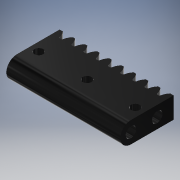
# Autodesk Inventor part: GA04
Saved by Autodesk Inventor 2017 (Build 210142000, 142)
## iProperties
Created: 2018-10-24
Part Number: GA04
Material: ABS Plastic
Document SubType Name: Modeling
Designer: Dell
Density: 1.06 g/cm^3
Appearance: Smooth - Black
Author: Dell
Autodesk Inventor part; units mm, degrees
ref_plane "YZ Plane" through (0, 0, 0) normal (1, 0, 0) x (0, 1, 0)
ref_plane "XZ Plane" through (0, 0, 0) normal (0, 1, 0) x (-1, 0, 0)
ref_plane "XY Plane" through (0, 0, 0) normal (0, 0, 1) x (1, 0, 0)
sketch "Sketch1" plane through (0, 0, 0) normal (0, 0, 1) x (1, 0, 0)
  spline S0 degree 3 poles (-2.7752, 20.8158) (-2.7042, 20.7277) (-2.562, 20.5515) (-2.36, 20.2785) (-2.1667, 19.9993) (-1.9839, 19.7131) (-1.8126, 19.4198) (-1.654, 19.1195) (-1.5101, 18.8118) (-1.3833, 18.4967) (-1.2955, 18.2274) (-1.2397, 18.008) (-1.2095, 17.8408) (-1.1935, 17.6716) (-1.162, 17.5046) (-1.1186, 17.3404) (-1.0623, 17.18) (-0.9883, 17.0268) (-0.8958, 16.884) (-0.7836, 16.7557) (-0.6724, 16.6674) (-0.5769, 16.6065) (-0.4998, 16.5707) (-0.4208, 16.5391) (-0.3383, 16.5188) (-0.2547, 16.503) (-0.1414, 16.4982) (0, 16.5012) (0.1414, 16.4982) (0.2547, 16.503) (0.3383, 16.5188) (0.4208, 16.5391) (0.4998, 16.5707) (0.5769, 16.6065) (0.6724, 16.6674) (0.7836, 16.7557) (0.8958, 16.884) (0.9883, 17.0268) (1.0623, 17.18) (1.1186, 17.3404) (1.162, 17.5046) (1.1935, 17.6716) (1.2095, 17.8408) (1.2397, 18.008) (1.2955, 18.2274) (1.3833, 18.4967) (1.5101, 18.8118) (1.654, 19.1195) (1.8126, 19.4198) (1.9839, 19.7131) (2.1667, 19.9993) (2.36, 20.2785) (2.562, 20.5515) (2.7042, 20.7277) (2.7752, 20.8158) knots 0 0 0 0 0.033953 0.067907 0.10186 0.135813 0.169766 0.203718 0.237669 0.271619 0.305565 0.322541 0.339512 0.356488 0.373464 0.390436 0.407409 0.424381 0.44135 0.458313 0.475267 0.483756 0.492243 0.500732 0.509218 0.517706 0.526192 0.543169 0.560147 0.568632 0.577121 0.585607 0.594095 0.602582 0.611072 0.628025 0.644989 0.661958 0.67893 0.695903 0.712875 0.729851 0.746827 0.763798 0.780774 0.81472 0.84867 0.882621 0.916573 0.950526 0.984479 1.018432 1.052385 1.086339 1.086339 1.086339 1.086339
  circle A0 centre (0, 0) radius 16.5 construction
  circle A1 centre (0, 0) radius 17.8542 construction
  circle A2 centre (0, 0) radius 19 construction
  circle A3 centre (0, 0) radius 21 construction
  line L0 (-2.7752, 20.8158) -> (2.7752, 20.8158)
  point P0 (-2.5639, 20.5501)
  point P1 (-2.3614, 20.2775)
  point P2 (-2.1684, 19.9981)
  point P3 (-1.9858, 19.7119)
  point P4 (-1.8147, 19.4186)
  point P5 (-1.6565, 19.1183)
  point P6 (-1.513, 18.8106)
  point P7 (-1.3869, 18.4953)
  point P8 (-1.2828, 18.1722)
  point P9 (-1.2417, 18.0075)
  point P10 (-1.2119, 17.8405)
  point P11 (-1.1909, 17.672)
  point P12 (-1.16, 17.5051)
  point P13 (-1.1164, 17.341)
  point P14 (-1.0594, 17.1812)
  point P15 (-0.9852, 17.0285)
  point P16 (-0.8925, 16.8864)
  point P17 (-0.78, 16.7594)
  point P18 (-0.648, 16.653)
  point P19 (-0.576, 16.6082)
  point P20 (-0.4995, 16.5714)
  point P21 (-0.4202, 16.541)
  point P22 (-0.3381, 16.5195)
  point P23 (-0.2545, 16.505)
  point P24 (-0.1698, 16.5)
  point P25 (0, 16.5)
  point P26 (0.1698, 16.5)
  point P27 (0.2545, 16.505)
  point P28 (0.3381, 16.5195)
  point P29 (0.4202, 16.541)
  point P30 (0.4995, 16.5714)
  point P31 (0.576, 16.6082)
  point P32 (0.648, 16.653)
  point P33 (0.78, 16.7594)
  point P34 (0.8925, 16.8864)
  point P35 (0.9852, 17.0285)
  point P36 (1.0594, 17.1812)
  point P37 (1.1164, 17.341)
  point P38 (1.16, 17.5051)
  point P39 (1.1909, 17.672)
  point P40 (1.2119, 17.8405)
  point P41 (1.2417, 18.0075)
  point P42 (1.2828, 18.1722)
  point P43 (1.3869, 18.4953)
  point P44 (1.513, 18.8106)
  point P45 (1.6565, 19.1183)
  point P46 (1.8147, 19.4186)
  point P47 (1.9858, 19.7119)
  point P48 (2.1684, 19.9981)
  point P49 (2.3614, 20.2775)
  point P50 (2.5639, 20.5501)
  constraints: 4 centre point, 2 end point, 2 point on circle, 1 horizontal, 111 other
sketch "Sketch2" plane through (0, 0, 0) normal (0, 0, 1) x (1, 0, 0)
  line L0 (32.5, 20.8158) -> (-32.5, 20.8158)
  line L1 (-32.5, 20.8158) -> (-32.5, 14.8158)
  line L2 (-32.5, 14.8158) -> (32.5, 14.8158)
  line L3 (32.5, 14.8158) -> (32.5, 20.8158)
  circle A0 centre (0, 0) radius 21 construction
  point P0 (0, 20.8158)
  point P1 (-2.7752, 20.8158)
  point P2 (2.7752, 20.8158)
  dimension "d2" = 6
  dimension "d3" = 65
  constraints: 8 end point, 2 parallel, 1 horizontal, 1 midpoint, 1 perpendicular, 1 point on line, 1 vertical alignment
  measures "d2" distance of L0.end L1.end
  measures "d3" distance of L1.end L2.end
extrude "Extrusion2" add sketch "Sketch2" along normal blind 10
extrude "Extrusion3" cut sketch "Sketch1" along normal blind 10
pattern_linear "Rectangular Pattern1" count 9 spacing 6.9446 along (-1, 0, 0) of "Extrusion3" first direction both ways yes
sketch "Sketch3" plane through (-32.5, 14.8158, 0) normal (-1, 0, 0) x (0, 0, 1)
  circle A0 centre (5, -3.3166) radius 6
  line L0 (0, 0) -> (10, 0) projected
  point P0 (0, -14.8158)
  point P1 (5, 0)
  dimension "d11" = 12
  constraints: 2 point on circle, 1 centre point, 1 midpoint, 1 vertical alignment
  measures "d11" diameter of A0
extrude "Extrusion4" add sketch "Sketch3" against normal blind 65 contours A0 L0 picked at (5.1596, -3.0992)
sketch "Sketch6" plane through (32.5, 20.8158, 10) normal (1, 0, 0) x (0, 0, -1)
  circle A0 centre (5, -24.3166) radius 6
  arc A1 (0, -6) -> (10, -6) centre (5, -9.3166) ccw projected
  line L0 (-1, -24.3166) -> (-1, -9.3166)
  line L1 (11, -9.3166) -> (11, -24.3166)
  arc A2 (-1, -9.3166) -> (11, -9.3166) centre (5, -9.3166) ccw
  point P0 (10, -20.8158)
  dimension "d21" = 15
  dimension "d22" = 12
  constraints: 6 point on circle, 4 end point, 4 tangent, 2 centre point, 1 concentric, 1 vertical alignment
  measures "d21" distance of A1.centre A0.centre
  measures "d22" diameter of A0
extrude "Extrusion6" add sketch "Sketch6" against normal blind 65
sketch "Sketch7" plane through (32.5, 20.8158, 10) normal (1, 0, 0) x (0, 0, -1)
  arc A0 (-1, -24.3166) -> (11, -24.3166) centre (5, -24.3166) ccw projected
  arc A1 (0, -6) -> (-1, -9.3166) centre (5, -9.3166) ccw projected
  circle A2 centre (5, -24.3166) radius 3
  circle A3 centre (5, -9.3166) radius 3
  point P0 (10, -20.8158)
  dimension "d25" = 6
  dimension "d26" = 6
  constraints: 2 centre point, 2 coincident
  measures "d25" diameter of A2
  measures "d26" diameter of A3
extrude "Extrusion7" cut sketch "Sketch7" against normal through all
sketch "Sketch8" plane through (32.5, -3.5008, 11) normal (0, 0, 1) x (1, 0, 0)
  line L0 (-65, 12) -> (-65, 18) projected
  line L1 (0, 18) -> (0, 12) projected
  line L2 (-65, -3) -> (-65, 3) projected
  line L3 (0, 3) -> (0, -3) projected
  circle A0 centre (-60, 7.5) radius 2.5
  circle A1 centre (-5, 7.5) radius 2.5
  circle A2 centre (-32.5, 7.5) radius 2.5
  line L4 (-5, 7.5) -> (-60, 7.5) construction
  line L5 (0, -6) -> (-65, -6) projected
  line L6 (-65, 3) -> (-65, 12)
  point P0 (-32.5, 3.5008)
  point P1 (-32.5, -6)
  point P2 (-65, 7.5)
  dimension "d29" = 5
  dimension "d30" = 5
  dimension "d31" = 5
  dimension "d32" = 55
  constraints: 4 end point, 3 centre point, 3 midpoint, 1 coincident, 1 horizontal, 1 horizontal alignment, 1 vertical, 1 vertical alignment
  measures "d29" diameter of A0
  measures "d30" diameter of A1
  measures "d31" diameter of A2
  measures "d32" distance of L4.start L4.end
extrude "Extrusion8" cut sketch "Sketch8" against normal through all
sketch "Sketch9" plane through (0, 0, 10) normal (0, 0, 1) x (1, 0, 0)
  spline S0 degree 3 poles (-25.0031, 20.8158) (-25.0741, 20.7277) (-25.2163, 20.5515) (-25.4183, 20.2785) (-25.6116, 19.9993) (-25.7944, 19.7131) (-25.9657, 19.4198) (-26.1243, 19.1195) (-26.2682, 18.8118) (-26.395, 18.4967) (-26.4828, 18.2274) (-26.5386, 18.008) (-26.5688, 17.8408) (-26.5848, 17.6716) (-26.6163, 17.5046) (-26.6597, 17.3404) (-26.716, 17.18) (-26.79, 17.0268) (-26.8825, 16.884) (-26.9947, 16.7557) (-27.1059, 16.6674) (-27.2014, 16.6065) (-27.2785, 16.5707) (-27.3575, 16.5391) (-27.44, 16.5188) (-27.5236, 16.503) (-27.6369, 16.4982) (-27.7783, 16.5012) (-27.9197, 16.4982) (-28.033, 16.503) (-28.1166, 16.5188) (-28.1991, 16.5391) (-28.2781, 16.5707) (-28.3552, 16.6065) (-28.4507, 16.6674) (-28.5619, 16.7557) (-28.6741, 16.884) (-28.7666, 17.0268) (-28.8406, 17.18) (-28.8969, 17.3404) (-28.9403, 17.5046) (-28.9718, 17.6716) (-28.9878, 17.8408) (-29.018, 18.008) (-29.0738, 18.2274) (-29.1616, 18.4967) (-29.2884, 18.8118) (-29.4323, 19.1195) (-29.5909, 19.4198) (-29.7622, 19.7131) (-29.945, 19.9993) (-30.1383, 20.2785) (-30.3403, 20.5515) (-30.4824, 20.7277) (-30.5535, 20.8158) knots 0 0 0 0 0.031255 0.06251 0.093765 0.125019 0.156273 0.187527 0.21878 0.250031 0.28128 0.296906 0.312529 0.328155 0.343782 0.359405 0.375029 0.390652 0.406273 0.421888 0.437494 0.445309 0.453121 0.460935 0.468747 0.476561 0.484372 0.5 0.515628 0.523439 0.531253 0.539065 0.546879 0.554691 0.562506 0.578112 0.593727 0.609348 0.624971 0.640595 0.656218 0.671845 0.687471 0.703094 0.71872 0.749969 0.78122 0.812473 0.843727 0.874981 0.906235 0.93749 0.968745 1 1 1 1 projected
  line L0 (-30.5535, 20.8158) -> (-32.5, 20.8158) projected
  line L1 (-32.5, 20.8158) -> (-32.5, 14.8158) projected
  line L2 (-32.5, 14.8158) -> (32.5, 14.8158) projected
  line L3 (32.5, 14.8158) -> (32.5, 20.8158) projected
  line L4 (32.5, 20.8158) -> (30.5535, 20.8158) projected
  spline S1 degree 3 poles (30.5535, 20.8158) (30.4824, 20.7277) (30.3403, 20.5515) (30.1383, 20.2785) (29.945, 19.9993) (29.7622, 19.7131) (29.5909, 19.4198) (29.4323, 19.1195) (29.2884, 18.8118) (29.1616, 18.4967) (29.0738, 18.2274) (29.018, 18.008) (28.9878, 17.8408) (28.9718, 17.6716) (28.9403, 17.5046) (28.8969, 17.3404) (28.8406, 17.18) (28.7666, 17.0268) (28.6741, 16.884) (28.5619, 16.7557) (28.4507, 16.6674) (28.3552, 16.6065) (28.2781, 16.5707) (28.1991, 16.5391) (28.1166, 16.5188) (28.033, 16.503) (27.9197, 16.4982) (27.7783, 16.5012) (27.6369, 16.4982) (27.5236, 16.503) (27.44, 16.5188) (27.3575, 16.5391) (27.2785, 16.5707) (27.2014, 16.6065) (27.1059, 16.6674) (26.9947, 16.7557) (26.8825, 16.884) (26.79, 17.0268) (26.716, 17.18) (26.6597, 17.3404) (26.6163, 17.5046) (26.5848, 17.6716) (26.5688, 17.8408) (26.5386, 18.008) (26.4828, 18.2274) (26.395, 18.4967) (26.2682, 18.8118) (26.1243, 19.1195) (25.9657, 19.4198) (25.7944, 19.7131) (25.6116, 19.9993) (25.4183, 20.2785) (25.2163, 20.5515) (25.0741, 20.7277) (25.0031, 20.8158) knots 0 0 0 0 0.031255 0.06251 0.093765 0.125019 0.156273 0.187527 0.21878 0.250031 0.28128 0.296906 0.312529 0.328155 0.343782 0.359405 0.375029 0.390652 0.406273 0.421888 0.437494 0.445309 0.453121 0.460935 0.468747 0.476561 0.484372 0.5 0.515628 0.523439 0.531253 0.539065 0.546879 0.554691 0.562506 0.578112 0.593727 0.609348 0.624971 0.640595 0.656218 0.671845 0.687471 0.703094 0.71872 0.749969 0.78122 0.812473 0.843727 0.874981 0.906235 0.93749 0.968745 1 1 1 1 projected
  line L5 (25.0031, 20.8158) -> (23.6089, 20.8158) projected
  spline S2 degree 3 poles (23.6089, 20.8158) (23.5379, 20.7277) (23.3958, 20.5515) (23.1937, 20.2785) (23.0004, 19.9993) (22.8177, 19.7131) (22.6463, 19.4198) (22.4877, 19.1195) (22.3438, 18.8118) (22.2171, 18.4967) (22.1292, 18.2274) (22.0734, 18.008) (22.0432, 17.8408) (22.0272, 17.6716) (21.9957, 17.5046) (21.9523, 17.3404) (21.896, 17.18) (21.822, 17.0268) (21.7296, 16.884) (21.6173, 16.7557) (21.5061, 16.6674) (21.4106, 16.6065) (21.3335, 16.5707) (21.2545, 16.5391) (21.172, 16.5188) (21.0884, 16.503) (20.9751, 16.4982) (20.8337, 16.5012) (20.6923, 16.4982) (20.579, 16.503) (20.4954, 16.5188) (20.4129, 16.5391) (20.3339, 16.5707) (20.2569, 16.6065) (20.1613, 16.6674) (20.0501, 16.7557) (19.9379, 16.884) (19.8454, 17.0268) (19.7714, 17.18) (19.7151, 17.3404) (19.6717, 17.5046) (19.6402, 17.6716) (19.6242, 17.8408) (19.594, 18.008) (19.5382, 18.2274) (19.4504, 18.4967) (19.3236, 18.8118) (19.1797, 19.1195) (19.0211, 19.4198) (18.8498, 19.7131) (18.667, 19.9993) (18.4738, 20.2785) (18.2717, 20.5515) (18.1296, 20.7277) (18.0585, 20.8158) knots 0 0 0 0 0.031255 0.06251 0.093765 0.125019 0.156273 0.187527 0.21878 0.250031 0.28128 0.296906 0.312529 0.328155 0.343782 0.359405 0.375029 0.390652 0.406273 0.421888 0.437494 0.445309 0.453121 0.460935 0.468747 0.476561 0.484372 0.5 0.515628 0.523439 0.531253 0.539065 0.546879 0.554691 0.562506 0.578112 0.593727 0.609348 0.624971 0.640595 0.656218 0.671845 0.687471 0.703094 0.71872 0.749969 0.78122 0.812473 0.843727 0.874981 0.906235 0.93749 0.968745 1 1 1 1 projected
  line L6 (18.0585, 20.8158) -> (16.6644, 20.8158) projected
  spline S3 degree 3 poles (16.6644, 20.8158) (16.5933, 20.7277) (16.4512, 20.5515) (16.2491, 20.2785) (16.0558, 19.9993) (15.8731, 19.7131) (15.7017, 19.4198) (15.5432, 19.1195) (15.3992, 18.8118) (15.2725, 18.4967) (15.1846, 18.2274) (15.1289, 18.008) (15.0986, 17.8408) (15.0827, 17.6716) (15.0512, 17.5046) (15.0077, 17.3404) (14.9515, 17.18) (14.8774, 17.0268) (14.785, 16.884) (14.6727, 16.7557) (14.5616, 16.6674) (14.466, 16.6065) (14.3889, 16.5707) (14.31, 16.5391) (14.2274, 16.5188) (14.1439, 16.503) (14.0306, 16.4982) (13.8891, 16.5012) (13.7477, 16.4982) (13.6344, 16.503) (13.5509, 16.5188) (13.4683, 16.5391) (13.3894, 16.5707) (13.3123, 16.6065) (13.2167, 16.6674) (13.1056, 16.7557) (12.9933, 16.884) (12.9008, 17.0268) (12.8268, 17.18) (12.7706, 17.3404) (12.7271, 17.5046) (12.6956, 17.6716) (12.6797, 17.8408) (12.6494, 18.008) (12.5936, 18.2274) (12.5058, 18.4967) (12.379, 18.8118) (12.2351, 19.1195) (12.0766, 19.4198) (11.9052, 19.7131) (11.7225, 19.9993) (11.5292, 20.2785) (11.3271, 20.5515) (11.185, 20.7277) (11.1139, 20.8158) knots 0 0 0 0 0.031255 0.06251 0.093765 0.125019 0.156273 0.187527 0.21878 0.250031 0.28128 0.296906 0.312529 0.328155 0.343782 0.359405 0.375029 0.390652 0.406273 0.421888 0.437494 0.445309 0.453121 0.460935 0.468747 0.476561 0.484372 0.5 0.515628 0.523439 0.531253 0.539065 0.546879 0.554691 0.562506 0.578112 0.593727 0.609348 0.624971 0.640595 0.656218 0.671845 0.687471 0.703094 0.71872 0.749969 0.78122 0.812473 0.843727 0.874981 0.906235 0.93749 0.968745 1 1 1 1 projected
  line L7 (11.1139, 20.8158) -> (9.7198, 20.8158) projected
  spline S4 degree 3 poles (9.7198, 20.8158) (9.6487, 20.7277) (9.5066, 20.5515) (9.3045, 20.2785) (9.1113, 19.9993) (8.9285, 19.7131) (8.7571, 19.4198) (8.5986, 19.1195) (8.4547, 18.8118) (8.3279, 18.4967) (8.2401, 18.2274) (8.1843, 18.008) (8.1541, 17.8408) (8.1381, 17.6716) (8.1066, 17.5046) (8.0632, 17.3404) (8.0069, 17.18) (7.9329, 17.0268) (7.8404, 16.884) (7.7282, 16.7557) (7.617, 16.6674) (7.5214, 16.6065) (7.4444, 16.5707) (7.3654, 16.5391) (7.2829, 16.5188) (7.1993, 16.503) (7.086, 16.4982) (6.9446, 16.5012) (6.8032, 16.4982) (6.6898, 16.503) (6.6063, 16.5188) (6.5237, 16.5391) (6.4448, 16.5707) (6.3677, 16.6065) (6.2722, 16.6674) (6.161, 16.7557) (6.0487, 16.884) (5.9563, 17.0268) (5.8822, 17.18) (5.826, 17.3404) (5.7826, 17.5046) (5.751, 17.6716) (5.7351, 17.8408) (5.7048, 18.008) (5.6491, 18.2274) (5.5612, 18.4967) (5.4345, 18.8118) (5.2905, 19.1195) (5.132, 19.4198) (4.9606, 19.7131) (4.7779, 19.9993) (4.5846, 20.2785) (4.3825, 20.5515) (4.2404, 20.7277) (4.1694, 20.8158) knots 0 0 0 0 0.031255 0.06251 0.093765 0.125019 0.156273 0.187527 0.21878 0.250031 0.28128 0.296906 0.312529 0.328155 0.343782 0.359405 0.375029 0.390652 0.406273 0.421888 0.437494 0.445309 0.453121 0.460935 0.468747 0.476561 0.484372 0.5 0.515628 0.523439 0.531253 0.539065 0.546879 0.554691 0.562506 0.578112 0.593727 0.609348 0.624971 0.640595 0.656218 0.671845 0.687471 0.703094 0.71872 0.749969 0.78122 0.812473 0.843727 0.874981 0.906235 0.93749 0.968745 1 1 1 1 projected
  line L8 (4.1694, 20.8158) -> (2.7752, 20.8158) projected
  spline S5 degree 3 poles (2.7752, 20.8158) (2.7042, 20.7277) (2.562, 20.5515) (2.36, 20.2785) (2.1667, 19.9993) (1.9839, 19.7131) (1.8126, 19.4198) (1.654, 19.1195) (1.5101, 18.8118) (1.3833, 18.4967) (1.2955, 18.2274) (1.2397, 18.008) (1.2095, 17.8408) (1.1935, 17.6716) (1.162, 17.5046) (1.1186, 17.3404) (1.0623, 17.18) (0.9883, 17.0268) (0.8958, 16.884) (0.7836, 16.7557) (0.6724, 16.6674) (0.5769, 16.6065) (0.4998, 16.5707) (0.4208, 16.5391) (0.3383, 16.5188) (0.2547, 16.503) (0.1414, 16.4982) (0, 16.5012) (-0.1414, 16.4982) (-0.2547, 16.503) (-0.3383, 16.5188) (-0.4208, 16.5391) (-0.4998, 16.5707) (-0.5769, 16.6065) (-0.6724, 16.6674) (-0.7836, 16.7557) (-0.8958, 16.884) (-0.9883, 17.0268) (-1.0623, 17.18) (-1.1186, 17.3404) (-1.162, 17.5046) (-1.1935, 17.6716) (-1.2095, 17.8408) (-1.2397, 18.008) (-1.2955, 18.2274) (-1.3833, 18.4967) (-1.5101, 18.8118) (-1.654, 19.1195) (-1.8126, 19.4198) (-1.9839, 19.7131) (-2.1667, 19.9993) (-2.36, 20.2785) (-2.562, 20.5515) (-2.7042, 20.7277) (-2.7752, 20.8158) knots 0 0 0 0 0.031255 0.06251 0.093765 0.125019 0.156273 0.187527 0.21878 0.250031 0.28128 0.296906 0.312529 0.328155 0.343782 0.359405 0.375029 0.390652 0.406273 0.421888 0.437494 0.445309 0.453121 0.460935 0.468747 0.476561 0.484372 0.5 0.515628 0.523439 0.531253 0.539065 0.546879 0.554691 0.562506 0.578112 0.593727 0.609348 0.624971 0.640595 0.656218 0.671845 0.687471 0.703094 0.71872 0.749969 0.78122 0.812473 0.843727 0.874981 0.906235 0.93749 0.968745 1 1 1 1 projected
  line L9 (-2.7752, 20.8158) -> (-4.1694, 20.8158) projected
  spline S6 degree 3 poles (-4.1694, 20.8158) (-4.2404, 20.7277) (-4.3825, 20.5515) (-4.5846, 20.2785) (-4.7779, 19.9993) (-4.9606, 19.7131) (-5.132, 19.4198) (-5.2905, 19.1195) (-5.4345, 18.8118) (-5.5612, 18.4967) (-5.6491, 18.2274) (-5.7048, 18.008) (-5.7351, 17.8408) (-5.751, 17.6716) (-5.7826, 17.5046) (-5.826, 17.3404) (-5.8822, 17.18) (-5.9563, 17.0268) (-6.0487, 16.884) (-6.161, 16.7557) (-6.2722, 16.6674) (-6.3677, 16.6065) (-6.4448, 16.5707) (-6.5237, 16.5391) (-6.6063, 16.5188) (-6.6898, 16.503) (-6.8032, 16.4982) (-6.9446, 16.5012) (-7.086, 16.4982) (-7.1993, 16.503) (-7.2829, 16.5188) (-7.3654, 16.5391) (-7.4444, 16.5707) (-7.5214, 16.6065) (-7.617, 16.6674) (-7.7282, 16.7557) (-7.8404, 16.884) (-7.9329, 17.0268) (-8.0069, 17.18) (-8.0632, 17.3404) (-8.1066, 17.5046) (-8.1381, 17.6716) (-8.1541, 17.8408) (-8.1843, 18.008) (-8.2401, 18.2274) (-8.3279, 18.4967) (-8.4547, 18.8118) (-8.5986, 19.1195) (-8.7571, 19.4198) (-8.9285, 19.7131) (-9.1113, 19.9993) (-9.3045, 20.2785) (-9.5066, 20.5515) (-9.6487, 20.7277) (-9.7198, 20.8158) knots 0 0 0 0 0.031255 0.06251 0.093765 0.125019 0.156273 0.187527 0.21878 0.250031 0.28128 0.296906 0.312529 0.328155 0.343782 0.359405 0.375029 0.390652 0.406273 0.421888 0.437494 0.445309 0.453121 0.460935 0.468747 0.476561 0.484372 0.5 0.515628 0.523439 0.531253 0.539065 0.546879 0.554691 0.562506 0.578112 0.593727 0.609348 0.624971 0.640595 0.656218 0.671845 0.687471 0.703094 0.71872 0.749969 0.78122 0.812473 0.843727 0.874981 0.906235 0.93749 0.968745 1 1 1 1 projected
  line L10 (-9.7198, 20.8158) -> (-11.1139, 20.8158) projected
  spline S7 degree 3 poles (-11.1139, 20.8158) (-11.185, 20.7277) (-11.3271, 20.5515) (-11.5292, 20.2785) (-11.7225, 19.9993) (-11.9052, 19.7131) (-12.0766, 19.4198) (-12.2351, 19.1195) (-12.379, 18.8118) (-12.5058, 18.4967) (-12.5936, 18.2274) (-12.6494, 18.008) (-12.6797, 17.8408) (-12.6956, 17.6716) (-12.7271, 17.5046) (-12.7706, 17.3404) (-12.8268, 17.18) (-12.9008, 17.0268) (-12.9933, 16.884) (-13.1056, 16.7557) (-13.2167, 16.6674) (-13.3123, 16.6065) (-13.3894, 16.5707) (-13.4683, 16.5391) (-13.5509, 16.5188) (-13.6344, 16.503) (-13.7477, 16.4982) (-13.8891, 16.5012) (-14.0306, 16.4982) (-14.1439, 16.503) (-14.2274, 16.5188) (-14.31, 16.5391) (-14.3889, 16.5707) (-14.466, 16.6065) (-14.5616, 16.6674) (-14.6727, 16.7557) (-14.785, 16.884) (-14.8774, 17.0268) (-14.9515, 17.18) (-15.0077, 17.3404) (-15.0512, 17.5046) (-15.0827, 17.6716) (-15.0986, 17.8408) (-15.1289, 18.008) (-15.1846, 18.2274) (-15.2725, 18.4967) (-15.3992, 18.8118) (-15.5432, 19.1195) (-15.7017, 19.4198) (-15.8731, 19.7131) (-16.0558, 19.9993) (-16.2491, 20.2785) (-16.4512, 20.5515) (-16.5933, 20.7277) (-16.6644, 20.8158) knots 0 0 0 0 0.031255 0.06251 0.093765 0.125019 0.156273 0.187527 0.21878 0.250031 0.28128 0.296906 0.312529 0.328155 0.343782 0.359405 0.375029 0.390652 0.406273 0.421888 0.437494 0.445309 0.453121 0.460935 0.468747 0.476561 0.484372 0.5 0.515628 0.523439 0.531253 0.539065 0.546879 0.554691 0.562506 0.578112 0.593727 0.609348 0.624971 0.640595 0.656218 0.671845 0.687471 0.703094 0.71872 0.749969 0.78122 0.812473 0.843727 0.874981 0.906235 0.93749 0.968745 1 1 1 1 projected
  line L11 (-16.6644, 20.8158) -> (-18.0585, 20.8158) projected
  spline S8 degree 3 poles (-18.0585, 20.8158) (-18.1296, 20.7277) (-18.2717, 20.5515) (-18.4738, 20.2785) (-18.667, 19.9993) (-18.8498, 19.7131) (-19.0211, 19.4198) (-19.1797, 19.1195) (-19.3236, 18.8118) (-19.4504, 18.4967) (-19.5382, 18.2274) (-19.594, 18.008) (-19.6242, 17.8408) (-19.6402, 17.6716) (-19.6717, 17.5046) (-19.7151, 17.3404) (-19.7714, 17.18) (-19.8454, 17.0268) (-19.9379, 16.884) (-20.0501, 16.7557) (-20.1613, 16.6674) (-20.2569, 16.6065) (-20.3339, 16.5707) (-20.4129, 16.5391) (-20.4954, 16.5188) (-20.579, 16.503) (-20.6923, 16.4982) (-20.8337, 16.5012) (-20.9751, 16.4982) (-21.0884, 16.503) (-21.172, 16.5188) (-21.2545, 16.5391) (-21.3335, 16.5707) (-21.4106, 16.6065) (-21.5061, 16.6674) (-21.6173, 16.7557) (-21.7296, 16.884) (-21.822, 17.0268) (-21.896, 17.18) (-21.9523, 17.3404) (-21.9957, 17.5046) (-22.0272, 17.6716) (-22.0432, 17.8408) (-22.0734, 18.008) (-22.1292, 18.2274) (-22.2171, 18.4967) (-22.3438, 18.8118) (-22.4877, 19.1195) (-22.6463, 19.4198) (-22.8177, 19.7131) (-23.0004, 19.9993) (-23.1937, 20.2785) (-23.3958, 20.5515) (-23.5379, 20.7277) (-23.6089, 20.8158) knots 0 0 0 0 0.031255 0.06251 0.093765 0.125019 0.156273 0.187527 0.21878 0.250031 0.28128 0.296906 0.312529 0.328155 0.343782 0.359405 0.375029 0.390652 0.406273 0.421888 0.437494 0.445309 0.453121 0.460935 0.468747 0.476561 0.484372 0.5 0.515628 0.523439 0.531253 0.539065 0.546879 0.554691 0.562506 0.578112 0.593727 0.609348 0.624971 0.640595 0.656218 0.671845 0.687471 0.703094 0.71872 0.749969 0.78122 0.812473 0.843727 0.874981 0.906235 0.93749 0.968745 1 1 1 1 projected
  line L12 (-23.6089, 20.8158) -> (-25.0031, 20.8158) projected
  line L13 (-32.5, 20.8158) -> (-32.5, 14.8158) projected
  line L14 (32.5, 8.4992) -> (-32.5, 8.4992) projected
  line L15 (-32.5, 14.8158) -> (32.5, 14.8158)
  line L16 (32.5, 14.8158) -> (32.5, 8.4992)
  line L17 (32.5, 8.4992) -> (-32.5, 8.4992)
  line L18 (-32.5, 8.4992) -> (-32.5, 14.8158)
  line L19 (32.5, 11.4992) -> (32.5, -3.5008) projected
  point P0 (0, 0)
  constraints: 9 horizontal alignment, 8 end point, 2 parallel, 2 point on line, 1 horizontal, 1 perpendicular
extrude "Extrusion9" add sketch "Sketch9" along normal blind 1
sketch "Sketch10" plane through (0, 0, 0) normal (0, 0, -1) x (-1, 0, 0)
  line L0 (32.5, 20.8158) -> (32.5, -3.5008) projected
  line L1 (-32.5, -3.5008) -> (32.5, -3.5008) projected
  line L2 (-32.5, 20.8158) -> (-32.5, -3.5008) projected
  line L3 (-32.5, 20.8158) -> (-30.5535, 20.8158) projected
  spline S0 degree 3 poles (-30.5535, 20.8158) (-30.4824, 20.7277) (-30.3403, 20.5515) (-30.1383, 20.2785) (-29.945, 19.9993) (-29.7622, 19.7131) (-29.5909, 19.4198) (-29.4323, 19.1195) (-29.2884, 18.8118) (-29.1616, 18.4967) (-29.0738, 18.2274) (-29.018, 18.008) (-28.9878, 17.8408) (-28.9718, 17.6716) (-28.9403, 17.5046) (-28.8969, 17.3404) (-28.8406, 17.18) (-28.7666, 17.0268) (-28.6741, 16.884) (-28.5619, 16.7557) (-28.4507, 16.6674) (-28.3552, 16.6065) (-28.2781, 16.5707) (-28.1991, 16.5391) (-28.1166, 16.5188) (-28.033, 16.503) (-27.9197, 16.4982) (-27.7783, 16.5012) (-27.6369, 16.4982) (-27.5236, 16.503) (-27.44, 16.5188) (-27.3575, 16.5391) (-27.2785, 16.5707) (-27.2014, 16.6065) (-27.1059, 16.6674) (-26.9947, 16.7557) (-26.8825, 16.884) (-26.79, 17.0268) (-26.716, 17.18) (-26.6597, 17.3404) (-26.6163, 17.5046) (-26.5848, 17.6716) (-26.5688, 17.8408) (-26.5386, 18.008) (-26.4828, 18.2274) (-26.395, 18.4967) (-26.2682, 18.8118) (-26.1243, 19.1195) (-25.9657, 19.4198) (-25.7944, 19.7131) (-25.6116, 19.9993) (-25.4183, 20.2785) (-25.2163, 20.5515) (-25.0741, 20.7277) (-25.0031, 20.8158) knots 0 0 0 0 0.031255 0.06251 0.093765 0.125019 0.156273 0.187527 0.21878 0.250031 0.28128 0.296906 0.312529 0.328155 0.343782 0.359405 0.375029 0.390652 0.406273 0.421888 0.437494 0.445309 0.453121 0.460935 0.468747 0.476561 0.484372 0.5 0.515628 0.523439 0.531253 0.539065 0.546879 0.554691 0.562506 0.578112 0.593727 0.609348 0.624971 0.640595 0.656218 0.671845 0.687471 0.703094 0.71872 0.749969 0.78122 0.812473 0.843727 0.874981 0.906235 0.93749 0.968745 1 1 1 1 projected
  line L4 (-25.0031, 20.8158) -> (-23.6089, 20.8158) projected
  spline S1 degree 3 poles (-23.6089, 20.8158) (-23.5379, 20.7277) (-23.3958, 20.5515) (-23.1937, 20.2785) (-23.0004, 19.9993) (-22.8177, 19.7131) (-22.6463, 19.4198) (-22.4877, 19.1195) (-22.3438, 18.8118) (-22.2171, 18.4967) (-22.1292, 18.2274) (-22.0734, 18.008) (-22.0432, 17.8408) (-22.0272, 17.6716) (-21.9957, 17.5046) (-21.9523, 17.3404) (-21.896, 17.18) (-21.822, 17.0268) (-21.7296, 16.884) (-21.6173, 16.7557) (-21.5061, 16.6674) (-21.4106, 16.6065) (-21.3335, 16.5707) (-21.2545, 16.5391) (-21.172, 16.5188) (-21.0884, 16.503) (-20.9751, 16.4982) (-20.8337, 16.5012) (-20.6923, 16.4982) (-20.579, 16.503) (-20.4954, 16.5188) (-20.4129, 16.5391) (-20.3339, 16.5707) (-20.2569, 16.6065) (-20.1613, 16.6674) (-20.0501, 16.7557) (-19.9379, 16.884) (-19.8454, 17.0268) (-19.7714, 17.18) (-19.7151, 17.3404) (-19.6717, 17.5046) (-19.6402, 17.6716) (-19.6242, 17.8408) (-19.594, 18.008) (-19.5382, 18.2274) (-19.4504, 18.4967) (-19.3236, 18.8118) (-19.1797, 19.1195) (-19.0211, 19.4198) (-18.8498, 19.7131) (-18.667, 19.9993) (-18.4738, 20.2785) (-18.2717, 20.5515) (-18.1296, 20.7277) (-18.0585, 20.8158) knots 0 0 0 0 0.031255 0.06251 0.093765 0.125019 0.156273 0.187527 0.21878 0.250031 0.28128 0.296906 0.312529 0.328155 0.343782 0.359405 0.375029 0.390652 0.406273 0.421888 0.437494 0.445309 0.453121 0.460935 0.468747 0.476561 0.484372 0.5 0.515628 0.523439 0.531253 0.539065 0.546879 0.554691 0.562506 0.578112 0.593727 0.609348 0.624971 0.640595 0.656218 0.671845 0.687471 0.703094 0.71872 0.749969 0.78122 0.812473 0.843727 0.874981 0.906235 0.93749 0.968745 1 1 1 1 projected
  line L5 (-18.0585, 20.8158) -> (-16.6644, 20.8158) projected
  spline S2 degree 3 poles (-16.6644, 20.8158) (-16.5933, 20.7277) (-16.4512, 20.5515) (-16.2491, 20.2785) (-16.0558, 19.9993) (-15.8731, 19.7131) (-15.7017, 19.4198) (-15.5432, 19.1195) (-15.3992, 18.8118) (-15.2725, 18.4967) (-15.1846, 18.2274) (-15.1289, 18.008) (-15.0986, 17.8408) (-15.0827, 17.6716) (-15.0512, 17.5046) (-15.0077, 17.3404) (-14.9515, 17.18) (-14.8774, 17.0268) (-14.785, 16.884) (-14.6727, 16.7557) (-14.5616, 16.6674) (-14.466, 16.6065) (-14.3889, 16.5707) (-14.31, 16.5391) (-14.2274, 16.5188) (-14.1439, 16.503) (-14.0306, 16.4982) (-13.8891, 16.5012) (-13.7477, 16.4982) (-13.6344, 16.503) (-13.5509, 16.5188) (-13.4683, 16.5391) (-13.3894, 16.5707) (-13.3123, 16.6065) (-13.2167, 16.6674) (-13.1056, 16.7557) (-12.9933, 16.884) (-12.9008, 17.0268) (-12.8268, 17.18) (-12.7706, 17.3404) (-12.7271, 17.5046) (-12.6956, 17.6716) (-12.6797, 17.8408) (-12.6494, 18.008) (-12.5936, 18.2274) (-12.5058, 18.4967) (-12.379, 18.8118) (-12.2351, 19.1195) (-12.0766, 19.4198) (-11.9052, 19.7131) (-11.7225, 19.9993) (-11.5292, 20.2785) (-11.3271, 20.5515) (-11.185, 20.7277) (-11.1139, 20.8158) knots 0 0 0 0 0.031255 0.06251 0.093765 0.125019 0.156273 0.187527 0.21878 0.250031 0.28128 0.296906 0.312529 0.328155 0.343782 0.359405 0.375029 0.390652 0.406273 0.421888 0.437494 0.445309 0.453121 0.460935 0.468747 0.476561 0.484372 0.5 0.515628 0.523439 0.531253 0.539065 0.546879 0.554691 0.562506 0.578112 0.593727 0.609348 0.624971 0.640595 0.656218 0.671845 0.687471 0.703094 0.71872 0.749969 0.78122 0.812473 0.843727 0.874981 0.906235 0.93749 0.968745 1 1 1 1 projected
  line L6 (-11.1139, 20.8158) -> (-9.7198, 20.8158) projected
  spline S3 degree 3 poles (-9.7198, 20.8158) (-9.6487, 20.7277) (-9.5066, 20.5515) (-9.3045, 20.2785) (-9.1113, 19.9993) (-8.9285, 19.7131) (-8.7571, 19.4198) (-8.5986, 19.1195) (-8.4547, 18.8118) (-8.3279, 18.4967) (-8.2401, 18.2274) (-8.1843, 18.008) (-8.1541, 17.8408) (-8.1381, 17.6716) (-8.1066, 17.5046) (-8.0632, 17.3404) (-8.0069, 17.18) (-7.9329, 17.0268) (-7.8404, 16.884) (-7.7282, 16.7557) (-7.617, 16.6674) (-7.5214, 16.6065) (-7.4444, 16.5707) (-7.3654, 16.5391) (-7.2829, 16.5188) (-7.1993, 16.503) (-7.086, 16.4982) (-6.9446, 16.5012) (-6.8032, 16.4982) (-6.6898, 16.503) (-6.6063, 16.5188) (-6.5237, 16.5391) (-6.4448, 16.5707) (-6.3677, 16.6065) (-6.2722, 16.6674) (-6.161, 16.7557) (-6.0487, 16.884) (-5.9563, 17.0268) (-5.8822, 17.18) (-5.826, 17.3404) (-5.7826, 17.5046) (-5.751, 17.6716) (-5.7351, 17.8408) (-5.7048, 18.008) (-5.6491, 18.2274) (-5.5612, 18.4967) (-5.4345, 18.8118) (-5.2905, 19.1195) (-5.132, 19.4198) (-4.9606, 19.7131) (-4.7779, 19.9993) (-4.5846, 20.2785) (-4.3825, 20.5515) (-4.2404, 20.7277) (-4.1694, 20.8158) knots 0 0 0 0 0.031255 0.06251 0.093765 0.125019 0.156273 0.187527 0.21878 0.250031 0.28128 0.296906 0.312529 0.328155 0.343782 0.359405 0.375029 0.390652 0.406273 0.421888 0.437494 0.445309 0.453121 0.460935 0.468747 0.476561 0.484372 0.5 0.515628 0.523439 0.531253 0.539065 0.546879 0.554691 0.562506 0.578112 0.593727 0.609348 0.624971 0.640595 0.656218 0.671845 0.687471 0.703094 0.71872 0.749969 0.78122 0.812473 0.843727 0.874981 0.906235 0.93749 0.968745 1 1 1 1 projected
  line L7 (-4.1694, 20.8158) -> (-2.7752, 20.8158) projected
  spline S4 degree 3 poles (-2.7752, 20.8158) (-2.7042, 20.7277) (-2.562, 20.5515) (-2.36, 20.2785) (-2.1667, 19.9993) (-1.9839, 19.7131) (-1.8126, 19.4198) (-1.654, 19.1195) (-1.5101, 18.8118) (-1.3833, 18.4967) (-1.2955, 18.2274) (-1.2397, 18.008) (-1.2095, 17.8408) (-1.1935, 17.6716) (-1.162, 17.5046) (-1.1186, 17.3404) (-1.0623, 17.18) (-0.9883, 17.0268) (-0.8958, 16.884) (-0.7836, 16.7557) (-0.6724, 16.6674) (-0.5769, 16.6065) (-0.4998, 16.5707) (-0.4208, 16.5391) (-0.3383, 16.5188) (-0.2547, 16.503) (-0.1414, 16.4982) (0, 16.5012) (0.1414, 16.4982) (0.2547, 16.503) (0.3383, 16.5188) (0.4208, 16.5391) (0.4998, 16.5707) (0.5769, 16.6065) (0.6724, 16.6674) (0.7836, 16.7557) (0.8958, 16.884) (0.9883, 17.0268) (1.0623, 17.18) (1.1186, 17.3404) (1.162, 17.5046) (1.1935, 17.6716) (1.2095, 17.8408) (1.2397, 18.008) (1.2955, 18.2274) (1.3833, 18.4967) (1.5101, 18.8118) (1.654, 19.1195) (1.8126, 19.4198) (1.9839, 19.7131) (2.1667, 19.9993) (2.36, 20.2785) (2.562, 20.5515) (2.7042, 20.7277) (2.7752, 20.8158) knots 0 0 0 0 0.031255 0.06251 0.093765 0.125019 0.156273 0.187527 0.21878 0.250031 0.28128 0.296906 0.312529 0.328155 0.343782 0.359405 0.375029 0.390652 0.406273 0.421888 0.437494 0.445309 0.453121 0.460935 0.468747 0.476561 0.484372 0.5 0.515628 0.523439 0.531253 0.539065 0.546879 0.554691 0.562506 0.578112 0.593727 0.609348 0.624971 0.640595 0.656218 0.671845 0.687471 0.703094 0.71872 0.749969 0.78122 0.812473 0.843727 0.874981 0.906235 0.93749 0.968745 1 1 1 1 projected
  line L8 (2.7752, 20.8158) -> (4.1694, 20.8158) projected
  spline S5 degree 3 poles (4.1694, 20.8158) (4.2404, 20.7277) (4.3825, 20.5515) (4.5846, 20.2785) (4.7779, 19.9993) (4.9606, 19.7131) (5.132, 19.4198) (5.2905, 19.1195) (5.4345, 18.8118) (5.5612, 18.4967) (5.6491, 18.2274) (5.7048, 18.008) (5.7351, 17.8408) (5.751, 17.6716) (5.7826, 17.5046) (5.826, 17.3404) (5.8822, 17.18) (5.9563, 17.0268) (6.0487, 16.884) (6.161, 16.7557) (6.2722, 16.6674) (6.3677, 16.6065) (6.4448, 16.5707) (6.5237, 16.5391) (6.6063, 16.5188) (6.6898, 16.503) (6.8032, 16.4982) (6.9446, 16.5012) (7.086, 16.4982) (7.1993, 16.503) (7.2829, 16.5188) (7.3654, 16.5391) (7.4444, 16.5707) (7.5214, 16.6065) (7.617, 16.6674) (7.7282, 16.7557) (7.8404, 16.884) (7.9329, 17.0268) (8.0069, 17.18) (8.0632, 17.3404) (8.1066, 17.5046) (8.1381, 17.6716) (8.1541, 17.8408) (8.1843, 18.008) (8.2401, 18.2274) (8.3279, 18.4967) (8.4547, 18.8118) (8.5986, 19.1195) (8.7571, 19.4198) (8.9285, 19.7131) (9.1113, 19.9993) (9.3045, 20.2785) (9.5066, 20.5515) (9.6487, 20.7277) (9.7198, 20.8158) knots 0 0 0 0 0.031255 0.06251 0.093765 0.125019 0.156273 0.187527 0.21878 0.250031 0.28128 0.296906 0.312529 0.328155 0.343782 0.359405 0.375029 0.390652 0.406273 0.421888 0.437494 0.445309 0.453121 0.460935 0.468747 0.476561 0.484372 0.5 0.515628 0.523439 0.531253 0.539065 0.546879 0.554691 0.562506 0.578112 0.593727 0.609348 0.624971 0.640595 0.656218 0.671845 0.687471 0.703094 0.71872 0.749969 0.78122 0.812473 0.843727 0.874981 0.906235 0.93749 0.968745 1 1 1 1 projected
  line L9 (9.7198, 20.8158) -> (11.1139, 20.8158) projected
  spline S6 degree 3 poles (11.1139, 20.8158) (11.185, 20.7277) (11.3271, 20.5515) (11.5292, 20.2785) (11.7225, 19.9993) (11.9052, 19.7131) (12.0766, 19.4198) (12.2351, 19.1195) (12.379, 18.8118) (12.5058, 18.4967) (12.5936, 18.2274) (12.6494, 18.008) (12.6797, 17.8408) (12.6956, 17.6716) (12.7271, 17.5046) (12.7706, 17.3404) (12.8268, 17.18) (12.9008, 17.0268) (12.9933, 16.884) (13.1056, 16.7557) (13.2167, 16.6674) (13.3123, 16.6065) (13.3894, 16.5707) (13.4683, 16.5391) (13.5509, 16.5188) (13.6344, 16.503) (13.7477, 16.4982) (13.8891, 16.5012) (14.0306, 16.4982) (14.1439, 16.503) (14.2274, 16.5188) (14.31, 16.5391) (14.3889, 16.5707) (14.466, 16.6065) (14.5616, 16.6674) (14.6727, 16.7557) (14.785, 16.884) (14.8774, 17.0268) (14.9515, 17.18) (15.0077, 17.3404) (15.0512, 17.5046) (15.0827, 17.6716) (15.0986, 17.8408) (15.1289, 18.008) (15.1846, 18.2274) (15.2725, 18.4967) (15.3992, 18.8118) (15.5432, 19.1195) (15.7017, 19.4198) (15.8731, 19.7131) (16.0558, 19.9993) (16.2491, 20.2785) (16.4512, 20.5515) (16.5933, 20.7277) (16.6644, 20.8158) knots 0 0 0 0 0.031255 0.06251 0.093765 0.125019 0.156273 0.187527 0.21878 0.250031 0.28128 0.296906 0.312529 0.328155 0.343782 0.359405 0.375029 0.390652 0.406273 0.421888 0.437494 0.445309 0.453121 0.460935 0.468747 0.476561 0.484372 0.5 0.515628 0.523439 0.531253 0.539065 0.546879 0.554691 0.562506 0.578112 0.593727 0.609348 0.624971 0.640595 0.656218 0.671845 0.687471 0.703094 0.71872 0.749969 0.78122 0.812473 0.843727 0.874981 0.906235 0.93749 0.968745 1 1 1 1 projected
  line L10 (16.6644, 20.8158) -> (18.0585, 20.8158) projected
  spline S7 degree 3 poles (18.0585, 20.8158) (18.1296, 20.7277) (18.2717, 20.5515) (18.4738, 20.2785) (18.667, 19.9993) (18.8498, 19.7131) (19.0211, 19.4198) (19.1797, 19.1195) (19.3236, 18.8118) (19.4504, 18.4967) (19.5382, 18.2274) (19.594, 18.008) (19.6242, 17.8408) (19.6402, 17.6716) (19.6717, 17.5046) (19.7151, 17.3404) (19.7714, 17.18) (19.8454, 17.0268) (19.9379, 16.884) (20.0501, 16.7557) (20.1613, 16.6674) (20.2569, 16.6065) (20.3339, 16.5707) (20.4129, 16.5391) (20.4954, 16.5188) (20.579, 16.503) (20.6923, 16.4982) (20.8337, 16.5012) (20.9751, 16.4982) (21.0884, 16.503) (21.172, 16.5188) (21.2545, 16.5391) (21.3335, 16.5707) (21.4106, 16.6065) (21.5061, 16.6674) (21.6173, 16.7557) (21.7296, 16.884) (21.822, 17.0268) (21.896, 17.18) (21.9523, 17.3404) (21.9957, 17.5046) (22.0272, 17.6716) (22.0432, 17.8408) (22.0734, 18.008) (22.1292, 18.2274) (22.2171, 18.4967) (22.3438, 18.8118) (22.4877, 19.1195) (22.6463, 19.4198) (22.8177, 19.7131) (23.0004, 19.9993) (23.1937, 20.2785) (23.3958, 20.5515) (23.5379, 20.7277) (23.6089, 20.8158) knots 0 0 0 0 0.031255 0.06251 0.093765 0.125019 0.156273 0.187527 0.21878 0.250031 0.28128 0.296906 0.312529 0.328155 0.343782 0.359405 0.375029 0.390652 0.406273 0.421888 0.437494 0.445309 0.453121 0.460935 0.468747 0.476561 0.484372 0.5 0.515628 0.523439 0.531253 0.539065 0.546879 0.554691 0.562506 0.578112 0.593727 0.609348 0.624971 0.640595 0.656218 0.671845 0.687471 0.703094 0.71872 0.749969 0.78122 0.812473 0.843727 0.874981 0.906235 0.93749 0.968745 1 1 1 1 projected
  line L11 (23.6089, 20.8158) -> (25.0031, 20.8158) projected
  spline S8 degree 3 poles (25.0031, 20.8158) (25.0741, 20.7277) (25.2163, 20.5515) (25.4183, 20.2785) (25.6116, 19.9993) (25.7944, 19.7131) (25.9657, 19.4198) (26.1243, 19.1195) (26.2682, 18.8118) (26.395, 18.4967) (26.4828, 18.2274) (26.5386, 18.008) (26.5688, 17.8408) (26.5848, 17.6716) (26.6163, 17.5046) (26.6597, 17.3404) (26.716, 17.18) (26.79, 17.0268) (26.8825, 16.884) (26.9947, 16.7557) (27.1059, 16.6674) (27.2014, 16.6065) (27.2785, 16.5707) (27.3575, 16.5391) (27.44, 16.5188) (27.5236, 16.503) (27.6369, 16.4982) (27.7783, 16.5012) (27.9197, 16.4982) (28.033, 16.503) (28.1166, 16.5188) (28.1991, 16.5391) (28.2781, 16.5707) (28.3552, 16.6065) (28.4507, 16.6674) (28.5619, 16.7557) (28.6741, 16.884) (28.7666, 17.0268) (28.8406, 17.18) (28.8969, 17.3404) (28.9403, 17.5046) (28.9718, 17.6716) (28.9878, 17.8408) (29.018, 18.008) (29.0738, 18.2274) (29.1616, 18.4967) (29.2884, 18.8118) (29.4323, 19.1195) (29.5909, 19.4198) (29.7622, 19.7131) (29.945, 19.9993) (30.1383, 20.2785) (30.3403, 20.5515) (30.4824, 20.7277) (30.5535, 20.8158) knots 0 0 0 0 0.031255 0.06251 0.093765 0.125019 0.156273 0.187527 0.21878 0.250031 0.28128 0.296906 0.312529 0.328155 0.343782 0.359405 0.375029 0.390652 0.406273 0.421888 0.437494 0.445309 0.453121 0.460935 0.468747 0.476561 0.484372 0.5 0.515628 0.523439 0.531253 0.539065 0.546879 0.554691 0.562506 0.578112 0.593727 0.609348 0.624971 0.640595 0.656218 0.671845 0.687471 0.703094 0.71872 0.749969 0.78122 0.812473 0.843727 0.874981 0.906235 0.93749 0.968745 1 1 1 1 projected
  line L12 (30.5535, 20.8158) -> (32.5, 20.8158) projected
  circle A0 centre (0, 3.9992) radius 2.5 projected
  circle A1 centre (27.5, 3.9992) radius 2.5 projected
  circle A2 centre (-27.5, 3.9992) radius 2.5 projected
  point P0 (0, 0)
  constraints: 9 horizontal alignment
extrude "Extrusion10" add sketch "Sketch10" along normal blind 1
equation "\"Module\" = 2"
equation "\"PressureAngle\" = 20deg"
equation "\"UnitProfileClearance\" = 0.25"
equation "\"UnitRoundRadius\" = 0.35"
equation "\"HeadDiameter\" = 42"
equation "\"RootDiameter\" = 33"
equation "\"BaseDiameter\" = 35.70832"
equation "\"PitchDiameter\" = 38"
equation "\"HelixAngle\" = 0"
equation "\"UnitCorrection\" = 0"
equation "\"UnitAddendumModification\" = 0"
equation "\"CircularPitch\" = 6.283185"
equation "\"UnitBacklashShift\" = 0"
equation "\"TotalToolShift\" = 0"
equation "\"IsInternal\" = 0"
body "Solid2"
